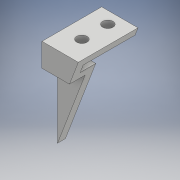
# Autodesk Inventor part: Side control right
Saved by Autodesk Inventor 2018 (Build 220112000, 112)
## iProperties
Created: 2019-11-10
Part Number: Side control right
Material: Типовые
Document SubType Name: Modeling
Designer: cosko
Density: 1 g/cm^3
Appearance: По умолчанию
Author: cosko
Autodesk Inventor part; units mm, degrees
ref_plane "YZ Plane" through (0, 0, 0) normal (1, 0, 0) x (0, 1, 0)
ref_plane "XZ Plane" through (0, 0, 0) normal (0, 1, 0) x (-1, 0, 0)
ref_plane "XY Plane" through (0, 0, 0) normal (0, 0, 1) x (1, 0, 0)
sketch "Эскиз1" plane through (0, 0, 0) normal (0, 0, 1) x (1, 0, 0)
  line L0 (-7, -11.5) -> (7, -11.5)
  line L1 (7, -11.5) -> (7, 11.5)
  line L2 (7, 11.5) -> (-7, 11.5)
  line L3 (-7, 11.5) -> (-7, -11.5)
  line L4 (-7, -11.5) -> (7, 11.5) construction
  line L5 (7, -11.5) -> (-7, 11.5) construction
  point P0 (0, 0)
  dimension "d0" = 14
  dimension "d1" = 23
  constraints: 12 end point, 2 midpoint, 2 parallel, 1 horizontal, 1 perpendicular
  measures "d0" distance of L2.end L1.end
  measures "d1" distance of L1.end L0.end
extrude "Выдавливание1" add sketch "Эскиз1" along normal blind 3
sketch "Эскиз2" plane through (0, 0, 0) normal (0, 0, -1) x (-1, 0, 0)
  line L0 (7, -11.5) -> (-7, -11.5) projected
  line L1 (7, 11.5) -> (7, -11.5) projected
  line L2 (-7, 11.5) -> (7, 11.5) projected
  line L3 (-7, -11.5) -> (-7, 11.5) projected
  line L4 (7, -11.5) -> (7, -8.5)
  line L5 (7, 11.5) -> (7, -11.5) construction
  line L6 (7, -11.5) -> (-7, -11.5) projected
  line L7 (7, -8.5) -> (-7, -8.5)
  line L8 (-7, -8.5) -> (-7, -11.5)
  line L9 (-7, -11.5) -> (7, -11.5)
  line L10 (7, -11.5) -> (7, -8.5)
  point P0 (0, 0)
  dimension "d4" = 3
  constraints: 10 end point, 2 parallel, 1 horizontal, 1 perpendicular, 1 point on line
  measures "d4" distance of L0.start L4.end
extrude "Выдавливание2" add sketch "Эскиз2" along normal blind 6 contours L0 L3 L7 L1
sketch "Эскиз3" plane through (-7, -8.5, 0) normal (0, 1, 0) x (1, 0, 0)
  line L0 (14, 6) -> (0, 6) projected
  line L1 (14, 0) -> (0, 0) projected
  line L2 (14, 0) -> (14, 6) projected
  line L3 (0, 6) -> (14, 6) projected
  line L4 (0, 0) -> (0, 6) projected
  line L5 (14, 6) -> (14, 3) construction
  line L6 (14, 0) -> (14, 6) construction
  line L7 (14, 3) -> (0, 3)
  line L8 (0, 3) -> (0, 6)
  line L9 (0, 6) -> (14, 6)
  line L10 (14, 6) -> (14, 3)
  point P0 (7, 0)
  dimension "d7" = 3
  constraints: 10 end point, 2 parallel, 1 horizontal, 1 midpoint, 1 perpendicular
  measures "d7" distance of L2.end L5.end
extrude "Выдавливание3" add sketch "Эскиз3" along normal blind 6 contours L2 L7 L4 L0
sketch "Эскиз4" plane through (0, 0, -6) normal (0, 0, -1) x (-1, 0, 0)
  line L0 (-7, -11.5) -> (7, -11.5) projected
  line L1 (7, -11.5) -> (7, -2.5) projected
  line L2 (-7, -2.5) -> (7, -2.5) projected
  line L3 (-7, -11.5) -> (-7, -2.5) projected
  line L4 (-7, -2.5) -> (7, -2.5) construction
  line L5 (-7, -2.5) -> (-7, -5.5) construction
  line L6 (-7, -5.5) -> (7, -5.5)
  line L7 (7, -5.5) -> (7, -2.5)
  line L8 (7, -2.5) -> (-7, -2.5)
  line L9 (-7, -2.5) -> (-7, -5.5)
  point P0 (0, 0)
  dimension "d10" = 3
  constraints: 10 end point, 2 parallel, 1 horizontal, 1 perpendicular, 1 point on line
  measures "d10" distance of L2.start L5.end
extrude "Выдавливание4" add sketch "Эскиз4" along normal blind 28 contours L3 L2 L1 L6
sketch "Эскиз6" plane through (0, 0, 3) normal (0, 0, 1) x (1, 0, 0)
  line L0 (-7, -11.5) -> (7, -11.5) projected
  line L1 (7, -11.5) -> (7, 11.5) projected
  line L2 (7, 11.5) -> (-7, 11.5) projected
  line L3 (-7, 0) -> (7, 0) construction
  line L4 (7, -8.5) -> (7, 11.5) construction
  line L5 (7, 11.5) -> (-7, 11.5) construction
  line L6 (0, 11.5) -> (0, -11.5) construction
  line L7 (0, 0) -> (0, 11.5) construction
  line L8 (0, 5.75) -> (-7, 5.75) construction
  line L9 (-7, 10) -> (-7, -10) construction
  line L10 (0, 5.75) -> (7, 5.75) construction
  line L11 (0, -11.5) -> (0, 0) construction
  line L12 (0, -5.75) -> (7, -5.75) construction
  line L13 (-7, 11.5) -> (-7, -11.5) projected
  line L14 (0, -11.5) -> (0, -3.131) construction
  line L15 (0, -3.131) -> (0, 6.869) construction
  circle A0 centre (0, -3.131) radius 2
  circle A1 centre (0, 6.869) radius 2
  point P0 (-5.8649, 10)
  dimension "d21" = 8.369
  dimension "d22" = 10
  dimension "d23" = 4
  dimension "d24" = 4
  constraints: 18 end point, 7 point on line, 3 midpoint, 3 perpendicular, 2 centre point, 2 coincident, 2 collinear, 3 other
  measures "d21" distance of L6.end L14.end
  measures "d22" distance of L14.end L15.end
  measures "d23" diameter of A0
  measures "d24" diameter of A1
extrude "Выдавливание6" cut sketch "Эскиз6" against normal up to next contours A0 | A1
sketch "Эскиз7" plane through (-7, -11.5, 3) normal (0, -1, 0) x (1, 0, 0)
  line L0 (14, -9) -> (14, 0) projected
  line L1 (0, 0) -> (14, 0) projected
  line L2 (0, 0) -> (0, -9) projected
  line L3 (14, -9) -> (0, -9) projected
  line L4 (0, -9) -> (14, -9) projected
  line L5 (0, -9) -> (0, -37) projected
  line L6 (14, -37) -> (0, -37) projected
  line L7 (14, -9) -> (14, -37) projected
  line L8 (0, 0) -> (14, 0) projected
  line L9 (0, -6) -> (0, -37) projected
  line L10 (14, 0) -> (0, -37)
  line L11 (0, -37) -> (14, -37)
  line L12 (14, -9) -> (14, 0) projected
  line L13 (14, 0) -> (14, -37)
  point P0 (7, -3)
  constraints: 6 end point, 1 collinear, 1 horizontal
extrude "Выдавливание7" cut sketch "Эскиз7" against normal blind 28 contours L3 L10 L0 | L7 L6 L10 L3
